Autodesk Fusion 360 part; units mm, degrees
note: some values were not read from the file. Set by a fixed rule: which sketch regions a step uses.
(part 3 of 3)
  line L1632 (31.5149, 83.2092) -> (31.5429, 83.2041)
  line L1633 (34.5916, 83.2488) -> (34.6161, 83.2634)
  line L1634 (34.3999, 83.2001) -> (34.3999, 83.1998)
  line L1635 (34.3999, 83.1998) -> (34.4284, 83.2009)
  line L1636 (34.7988, 83.5713) -> (34.7998, 83.5998)
  line L1637 (34.6396, 83.2796) -> (34.6618, 83.2976)
  line L1638 (31.5429, 83.2041) -> (31.5713, 83.2011)
  line L1639 (31.317, 83.3172) -> (31.3379, 83.2977)
  line L1640 (34.6618, 83.2976) -> (34.6827, 83.317)
  line L1641 (34.7509, 83.4082) -> (34.7637, 83.4337)
  line L1642 (31.5713, 83.2011) -> (31.5999, 83.2001)
  line L1643 (31.4337, 83.2362) -> (31.4601, 83.2253)
  line L1644 (34.4284, 83.2009) -> (34.4568, 83.2039)
  line L1645 (34.7907, 83.5148) -> (34.7958, 83.5429)
  line L1646 (31.4872, 83.2163) -> (31.5149, 83.2092)
  line L1647 (34.7836, 83.4872) -> (34.7907, 83.5148)
  line L1648 (31.2855, 86.2476) -> (31.268, 86.2237)
  line L1649 (34.4568, 83.2039) -> (34.4849, 83.209)
  line L1650 (34.6827, 83.317) -> (34.7022, 83.3379)
  line L1651 (34.5126, 83.2161) -> (34.5397, 83.2251)
  line L1652 (31.4082, 83.249) -> (31.4337, 83.2362)
  line L1653 (31.2488, 83.4083) -> (31.2634, 83.3838)
  line L1654 (31.4601, 83.2253) -> (31.4872, 83.2163)
  line L1655 (34.7201, 83.3601) -> (34.7364, 83.3836)
  line L1656 (34.7746, 83.4601) -> (34.7836, 83.4872)
  line L1657 (34.7022, 83.3379) -> (34.7201, 83.3601)
  line L1658 (31.3836, 83.2635) -> (31.4082, 83.249)
  line L1659 (31.1999, 86.0005) -> (31.1999, 86.0001)
  line L1660 (34.7022, 86.2623) -> (34.6827, 86.2832)
  line L1661 (31.2161, 83.4873) -> (31.2251, 83.4602)
  line L1662 (31.2251, 83.4602) -> (31.236, 83.4339)
  line L1663 (31.4223, 86.3588) -> (31.3962, 86.3446)
  line L1664 (11.2634, 83.3838) -> (11.2797, 83.3603)
  line L1665 (11.2976, 83.3381) -> (11.317, 83.3172)
  line L1666 (11.2161, 83.4873) -> (11.2251, 83.4602)
  line L1667 (14.7022, 86.2623) -> (14.6827, 86.2832)
  line L1668 (14.7958, 86.0573) -> (14.7907, 86.0854)
  line L1669 (11.4771, 86.381) -> (11.4493, 86.3709)
  line L1670 (11.2797, 83.3603) -> (11.2976, 83.3381)
  line L1671 (14.5397, 86.3751) -> (14.5126, 86.3841)
  line L1672 (14.566, 86.3642) -> (14.5397, 86.3751)
  line L1673 (14.7509, 86.192) -> (14.7364, 86.2166)
  line L1674 (14.6396, 86.3206) -> (14.6161, 86.3368)
  line L1675 (14.6161, 86.3368) -> (14.5916, 86.3514)
  line L1676 (14.6618, 86.3026) -> (14.6396, 86.3206)
  line L1677 (11.3254, 86.2913) -> (11.3046, 86.2702)
  line L1678 (11.4223, 86.3588) -> (11.3962, 86.3446)
  line L1679 (14.4568, 86.3963) -> (14.4284, 86.3993)
  line L1680 (14.7988, 86.0289) -> (14.7958, 86.0573)
  line L1681 (14.7836, 86.113) -> (14.7746, 86.1401)
  line L1682 (14.7998, 86.0004) -> (14.7988, 86.0289)
  line L1683 (11.3962, 86.3446) -> (11.3713, 86.3286)
  line L1684 (11.1999, 86.0005) -> (11.1999, 86.0001)
  line L1685 (11.3379, 83.2977) -> (11.3602, 83.2798)
  line L1686 (11.2043, 86.0594) -> (11.201, 86.0299)
  line L1687 (14.7637, 86.1665) -> (14.7509, 86.192)
  line L1688 (11.3713, 86.3286) -> (11.3477, 86.3108)
  line L1689 (14.4284, 86.3993) -> (14.3999, 86.4004)
  line L1690 (14.5126, 86.3841) -> (14.4849, 86.3912)
  line L1691 (14.5916, 86.3514) -> (14.566, 86.3642)
  line L1692 (14.6827, 86.2832) -> (14.6618, 86.3026)
  line L1693 (14.7201, 86.2401) -> (14.7022, 86.2623)
  line L1694 (14.3999, 83.2001) -> (14.3999, 83.1998)
  line L1695 (11.317, 83.3172) -> (11.3379, 83.2977)
  line L1696 (14.5916, 83.2488) -> (14.6161, 83.2634)
  line L1697 (14.7201, 83.3601) -> (14.7364, 83.3836)
  line L1698 (14.7958, 83.5429) -> (14.7988, 83.5713)
  line L1699 (14.6618, 83.2976) -> (14.6827, 83.317)
  line L1700 (11.2009, 83.5715) -> (11.2039, 83.5431)
  line L1701 (14.7998, 83.5998) -> (14.7998, 86.0004)
  line L1702 (14.7988, 83.5713) -> (14.7998, 83.5998)
  line L1703 (11.5713, 83.2011) -> (11.5999, 83.2001)
  line L1704 (11.4082, 83.249) -> (11.4337, 83.2362)
  line L1705 (11.2524, 86.1985) -> (11.2387, 86.1723)
  line L1706 (11.564, 86.3987) -> (11.5346, 86.395)
  line L1707 (11.4337, 83.2362) -> (11.4601, 83.2253)
  line L1708 (14.7509, 83.4082) -> (14.7637, 83.4337)
  line L1709 (11.236, 83.4339) -> (11.2488, 83.4083)
  line L1710 (14.6827, 83.317) -> (14.7022, 83.3379)
  line L1711 (11.3602, 83.2798) -> (11.3836, 83.2635)
  line L1712 (14.3999, 86.4002) -> (11.5999, 86.4002)
  line L1713 (11.5149, 83.2092) -> (11.5429, 83.2041)
  line L1714 (14.5397, 83.2251) -> (14.566, 83.236)
  line L1715 (11.4601, 83.2253) -> (11.4872, 83.2163)
  line L1716 (14.7836, 83.4872) -> (14.7907, 83.5148)
  line L1717 (11.2173, 86.1171) -> (11.2097, 86.0885)
  line L1718 (11.5999, 83.2001) -> (14.3999, 83.2001)
  line L1719 (11.2039, 83.5431) -> (11.209, 83.515)
  line L1720 (14.566, 83.236) -> (14.5916, 83.2488)
  line L1721 (11.1999, 86.0004) -> (11.1999, 86.0005)
  line L1722 (11.2488, 83.4083) -> (11.2634, 83.3838)
  line L1723 (11.2387, 86.1723) -> (11.227, 86.1451)
  line L1724 (14.4284, 83.2009) -> (14.4568, 83.2039)
  line L1725 (11.2251, 83.4602) -> (11.236, 83.4339)
  line L1726 (11.3477, 86.3108) -> (11.3254, 86.2913)
  line L1727 (14.6161, 83.2634) -> (14.6396, 83.2796)
  line L1728 (11.5429, 83.2041) -> (11.5713, 83.2011)
  line L1729 (11.268, 86.2237) -> (11.2524, 86.1985)
  line L1730 (11.1999, 83.6) -> (11.2009, 83.5715)
  line L1731 (11.3836, 83.2635) -> (11.4082, 83.249)
  line L1732 (11.201, 86.0299) -> (11.1999, 86.0004)
  line L1733 (14.7022, 83.3379) -> (14.7201, 83.3601)
  line L1734 (14.3999, 86.4004) -> (14.3999, 86.4002)
  line L1735 (11.5999, 86.4002) -> (11.5935, 86.4003)
  line L1736 (14.4849, 83.209) -> (14.5126, 83.2161)
  line L1737 (14.5126, 83.2161) -> (14.5397, 83.2251)
  line L1738 (11.3046, 86.2702) -> (11.2855, 86.2476)
  line L1739 (14.7907, 83.5148) -> (14.7958, 83.5429)
  line L1740 (14.4568, 83.2039) -> (14.4849, 83.209)
  line L1741 (14.6396, 83.2796) -> (14.6618, 83.2976)
  line L1742 (14.7637, 83.4337) -> (14.7746, 83.4601)
  line L1743 (11.4493, 86.3709) -> (11.4223, 86.3588)
  line L1744 (11.5346, 86.395) -> (11.5056, 86.3891)
  line L1745 (11.5056, 86.3891) -> (11.4771, 86.381)
  line L1746 (11.2097, 86.0885) -> (11.2043, 86.0594)
  line L1747 (11.227, 86.1451) -> (11.2173, 86.1171)
  line L1748 (14.3999, 83.1998) -> (14.4284, 83.2009)
  line L1749 (11.1999, 86.0001) -> (11.1999, 83.6)
  line L1750 (11.4872, 83.2163) -> (11.5149, 83.2092)
  line L1751 (14.7746, 83.4601) -> (14.7836, 83.4872)
  line L1752 (14.7364, 83.3836) -> (14.7509, 83.4082)
  line L1753 (11.2855, 86.2476) -> (11.268, 86.2237)
  line L1754 (11.209, 83.515) -> (11.2161, 83.4873)
  line L1755 (14.7364, 86.2166) -> (14.7201, 86.2401)
  line L1756 (11.5935, 86.4003) -> (11.564, 86.3987)
  line L1757 (14.7746, 86.1401) -> (14.7637, 86.1665)
  line L1758 (14.7907, 86.0854) -> (14.7836, 86.113)
  line L1759 (14.4849, 86.3912) -> (14.4568, 86.3963)
  circle A286 centre (73.2167, 97.5019) radius 0.5715
  circle A287 centre (73.2167, 94.9619) radius 0.5715
  circle A288 centre (70.6767, 94.9619) radius 0.5715
  circle A289 centre (70.6767, 97.5019) radius 0.5715
  circle A290 centre (2.7501, 82.0094) radius 0.1525
  circle A291 centre (4.1397, 72.1394) radius 0.1525
  circle A292 centre (55.3625, 4.8512) radius 0.1525
  circle A293 centre (83.4765, 37.5893) radius 0.1525
  circle A294 centre (84.9014, 37.0879) radius 0.1525
  circle A295 centre (85.5502, 48.3719) radius 0.1525
  circle A296 centre (1.2499, 56.5799) radius 0.1525
  circle A297 centre (1.2629, 36.6652) radius 0.1525
  circle A298 centre (1.2629, 17.0602) radius 0.1525
  circle A299 centre (15.4999, 3.6609) radius 0.1525
  circle A300 centre (82.4298, 9.7066) radius 0.1525
  circle A301 centre (81.87, 25.6347) radius 0.1525
  circle A302 centre (85.5502, 29.0599) radius 0.1525
  circle A303 centre (76.9604, 65.003) radius 0.1525
  circle A304 centre (84.3142, 65.0886) radius 0.1525
  circle A305 centre (55.4999, 94.2799) radius 0.1525
  circle A306 centre (71.8054, 89.6287) radius 0.1525
  circle A307 centre (28.4125, 5.746) radius 0.1525
  circle A308 centre (49.3993, 1.2499) radius 0.1525
  circle A309 centre (17.4168, 5.746) radius 0.1525
  circle A310 centre (1.59, 9.3917) radius 0.1525
  circle A311 centre (6.1252, 12.2731) radius 0.1525
  circle A312 centre (15.459, 4.683) radius 0.1525
  circle A313 centre (36.6005, 2.4468) radius 0.1525
  circle A314 centre (76.6005, 1.2499) radius 0.1525
  circle A315 centre (50.1026, 3.6355) radius 0.1525
  circle A316 centre (86.3874, 68.7488) radius 0.1525
  circle A317 centre (84.05, 69.3995) radius 0.1525
  line L1760 (-10.2, 110.2) -> (97.2, 110.2)
  line L1761 (97.2, 110.2) -> (97.2, -10.2)
  line L1762 (97.2, -10.2) -> (-10.2, -10.2)
  line L1763 (-10.2, -10.2) -> (-10.2, 110.2)
  constraint horizontal L1760
  constraint vertical L1761
  constraint horizontal L1762
  constraint vertical L1763
extrude "Extrude3" add sketch "PCB_hackpad_2026-02-28" 1 faces at (-4.0758, 13, -66.7333) along normal blind 3 separate body contours L0 L1 L2 L3 L200 L201 L202 L204 L205 L206 L207 L212 L213 L214 L215 L216 L217 L218 L220 L221 L222 | L3 L181 L202 L203 L216 L219 L220 L222 | L181 L200 L202 L222 | L181 L202 L203 L222 | L181 L216 L219 L220 | L181 L216 L218 L220 | L181 L200 L201 L222 | L181 L201 L203 L222 | L181 L217 L219 L220 | L181 L217 L218 L220 | L181 L201 L203 L204 L207 L213 L214 L217 L219 L220 L221 L222 | L204 L205 L206 L207 L221 L222 | L204 L207 L221 L222 | L213 L214 L220 L221 | L212 L213 L214 L215 L220 L221 | L36 L37 L38 L39 | L40 L41 L42 L43 | L44 L45 L46 L47 | L48 L49 L50 L51 | L52 L53 L54 L55 | L56 L57 L58 L59 | L60 L61 L62 L63 | L64 L65 L66 L67 | L68 L69 L70 L71 | L72 L73 L74 L75 | L76 L77 L78 L79 | L80 L81 L82 L83 | L84 L85 L86 L87 | L88 L89 L90 L91 | L92 L93 L94 L95 | L96 L97 L98 L99 A87 A169 | L99 A87 A169 A247 | L99 A87 A169 A247 | L99 A247 | L99 A247 | A0 | A1 | A2 | A3 | A4 | A5 | A6 | A7 | A8 | A9 | A10 | A11 | A12 | A13 | A14 | A15 | L101 L102 L103 L104 | L106 L107 L108 L109 | L111 L112 L113 L114 | L116 L117 L118 L119 | L121 L122 L123 L124 | L126 L127 L128 L129 | L131 L132 L133 L134 | L136 L137 L138 L139 | L141 L142 L143 L144 | L146 L147 L148 L149 | L151 L152 L153 L154 | L156 L157 L158 L159 | L161 L162 L163 L164 | L166 L167 L168 L169 | L171 L172 L173 L174 A268 | L173 A268 A304 | L173 A268 A304 | L173 A304 | L173 A304 | L176 L177 L178 L179 | L208 L209 L210 L211 | A16 A94 | A17 A95 | A18 A96 | A19 A97 | A20 A98 | A21 A99 | A22 A100 | A23 A101 | A24 A102 | A25 A103 | A26 A104 | A27 A105 | A28 A106 | A29 A107 | A30 A108 | A31 A109 | A32 A110 | A33 A111 | A34 A112 | A35 A113 | A36 A114 | A37 A115 | A38 A116 | A39 A117 | A40 A118 | A41 A119 | A42 A120 | A43 A121 | A44 A122 | A45 A123 | A46 A124 | A47 A125 | A48 A126 | A49 A127 | A50 A128 | A51 A129 | A52 A130 | A53 A131 | A54 A132 | A55 A133 | A56 A134 | A57 A135 | A58 A136 | A59 A137 | A60 A138 | A61 A139 | A62 A140 | A63 A141 | A64 A142 | A65 A143 | A66 A144 | A67 A145 | A68 A146 | A69 A147 | A70 A148 | A71 A149 | A72 A150 | A73 A151 | A74 A152 | A75 A153 | A76 A154 | A77 A155 | A78 A156 | A79 A157 | A80 A162 | A81 A163 | A82 A164 | A83 A165 | A84 A166 | A85 A167 | A86 A168 | A88 A170 | A89 A171 | A90 A172 | A91 A173 | A92 A174 | A93 A175 | A158 | A159 | A160 | A161 | A176 | A177 | A178 | A179 | A180 | A181 | A182 | A183 | A184 | A185 | A186 | A187 | A188 | A189 | A190 | A191 | A192 | A193 | A194 | A195 | A196 | A197 | A198 | A199 | A200 | A201 | A202 | A203 | A204 | A205 | A206 | A207 | A208 | A209 | A210 | A211 | A212 | A213 | A214 | A215 | A216 | A217 | A218 | A219 | A220 | A221 | A222 | A223 | A224 | A225 | A226 | A227 | A228 | A229 | A230 | A231 | A232 | A233 | A234 | A235 | A236 | A237 | A238 | A239 | A240 | A241 | A242 | A243 | A244 | A245 | A246 | A248 | A249 | A250 | A251 | A252 | A253 | A254 | A255 | A256 | A257 | A258 | A259 | A260 | A261 | A262 | A263 | A264 | A265 | A266 | A267 | A269 | A270 | A271 | A272 | A273 | A274 | A275 | A276 | A277 | A278 | A279 | A280 | A281 | A282 | A283 | A284 | A285 | L224 L225 L226 L227 L228 L229 L230 L231 L232 L233 L234 L236 L237 L238 L239 L240 L241 L242 L243 L244 L245 L246 L247 L248 L249 L250 L251 L252 L253 L254 L255 L256 L257 L258 L259 L260 L262 L263 L265 L266 L268 L269 L270 L271 L272 L273 L274 L275 L276 L277 L278 L279 L280 L281 L282 L283 L284 L285 L286 L287 L288 L289 L290 L291 L292 L293 L294 L295 L296 L297 L298 L299 L300 L301 L302 L303 L304 L305 L306 L307 L308 L309 L310 L311 L312 L313 L314 L315 L316 L317 L318 L319 | L320 L321 L322 L323 L324 L326 L327 L328 L329 L330 L331 L332 L333 L334 L335 L336 L337 L338 L339 L340 L341 L342 L343 L344 L345 L346 L347 L348 L349 L350 L351 L352 L353 L354 L355 L356 L357 L358 L359 L360 L361 L362 L363 L364 L365 L366 L367 L368 L369 L370 L371 L373 L374 L375 L376 L377 L378 L379 L380 L381 L382 L383 L384 L385 L386 L389 L390 L391 L392 L393 L394 L395 L396 L397 L398 L399 L400 L401 L402 L403 L404 L405 L406 L407 L408 L409 L410 L411 L412 L413 L414 L415 | L416 L417 L418 L419 L420 L421 L422 L423 L424 L425 L426 L428 L429 L431 L432 L433 L434 L435 L436 L437 L438 L439 L440 L441 L442 L443 L444 L445 L446 L447 L448 L449 L450 L451 L452 L453 L454 L455 L456 L457 L458 L459 L460 L461 L462 L463 L464 L465 L466 L468 L470 L471 L472 L473 L474 L475 L476 L477 L478 L479 L480 L481 L482 L483 L484 L485 L486 L487 L488 L489 L490 L491 L492 L493 L494 L495 L496 L497 L498 L499 L500 L501 L502 L503 L504 L505 L506 L507 L508 L509 L510 L511 | L512 L513 L514 L515 L516 L517 L518 L519 L520 L521 L522 L523 L524 L525 L526 L527 L528 L529 L530 L531 L532 L533 L534 L535 L536 L537 L538 L539 L540 L542 L543 L544 L545 L546 L547 L548 L549 L550 L551 L552 L553 L554 L555 L556 L557 L558 L559 L560 L561 L562 L563 L564 L565 L566 L567 L568 L569 L571 L572 L573 L574 L575 L576 L577 L578 L579 L580 L581 L582 L583 L584 L585 L586 L587 L589 L590 L591 L592 L593 L594 L595 L596 L598 L599 L600 L601 L602 L603 L604 L605 L606 L607 | L608 L609 L610 L611 L612 L613 L614 L615 L616 L617 L618 L619 L620 L621 L622 L623 L624 L625 L626 L627 L628 L629 L630 L631 L632 L633 L634 L636 L637 L638 L639 L640 L641 L642 L643 L644 L645 L647 L648 L649 L650 L651 L652 L654 L655 L656 L657 L658 L659 L660 L661 L662 L663 L664 L665 L666 L667 L668 L669 L670 L671 L672 L673 L674 L675 L676 L677 L678 L679 L680 L681 L683 L684 L685 L686 L687 L688 L689 L690 L691 L692 L693 L694 L695 L696 L697 L698 L699 L700 L701 L702 L703 | L704 L705 L706 L707 L708 L709 L710 L711 L712 L713 L714 L715 L716 L717 L718 L719 L720 L721 L722 L723 L724 L725 L726 L727 L729 L730 L731 L732 L733 L734 L735 L738 L739 L740 L741 L742 L743 L744 L745 L746 L747 L748 L749 L751 L752 L753 L754 L755 L756 L757 L758 L759 L760 L761 L762 L763 L764 L765 L766 L767 L768 L769 L770 L771 L772 L773 L774 L775 L776 L777 L778 L779 L780 L781 L782 L783 L784 L785 L786 L787 L788 L789 L790 L791 L792 L793 L794 L795 L796 L797 L798 L799 | L800 L801 L802 L803 L804 L805 L806 L807 L808 L809 L811 L812 L813 L814 L815 L816 L817 L818 L819 L820 L821 L822 L823 L824 L825 L826 L827 L828 L829 L830 L831 L832 L833 L834 L835 L836 L837 L838 L839 L840 L841 L842 L843 L844 L845 L846 L847 L848 L849 L850 L851 L852 L853 L854 L855 L856 L857 L858 L859 L860 L861 L862 L863 L865 L866 L867 L868 L869 L870 L871 L872 L873 L874 L875 L876 L877 L878 L879 L880 L881 L883 L884 L885 L886 L887 L888 L889 L890 L891 L892 L894 L895 | L896 L897 L898 L899 L900 L901 L902 L903 L904 L905 L906 L907 L908 L910 L911 L912 L913 L914 L915 L916 L917 L918 L919 L920 L921 L922 L924 L925 L926 L927 L928 L929 L930 L931 L932 L933 L934 L935 L936 L937 L938 L939 L940 L941 L942 L943 L944 L945 L946 L947 L948 L949 L950 L951 L952 L953 L954 L955 L956 L957 L958 L960 L961 L962 L963 L964 L965 L966 L967 L968 L969 L970 L971 L972 L974 L975 L976 L977 L978 L979 L980 L981 L982 L983 L984 L985 L986 L987 L988 L989 L990 L991 | L992 L993 L994 L995 L996 L997 L998 L999 L1000 L1001 L1002 L1003 L1004 L1005 L1006 L1007 L1008 L1009 L1010 L1011 L1012 L1013 L1014 L1015 L1016 L1018 L1019 L1020 L1021 L1022 L1023 L1024 L1026 L1027 L1029 L1030 L1031 L1032 L1033 L1034 L1035 L1036 L1037 L1038 L1039 L1040 L1041 L1042 L1044 L1045 L1046 L1047 L1048 L1049 L1050 L1051 L1052 L1053 L1054 L1055 L1056 L1057 L1058 L1059 L1060 L1061 L1062 L1063 L1064 L1065 L1066 L1067 L1068 L1069 L1070 L1071 L1072 L1073 L1074 L1075 L1076 L1077 L1078 L1079 L1080 L1081 L1082 L1083 L1084 L1085 L1086 L1087 | L1089 L1090 L1091 L1092 L1093 L1094 L1095 L1096 L1097 L1098 L1099 L1100 L1101 L1102 L1103 L1104 L1105 L1106 L1107 L1108 L1110 L1111 L1112 L1113 L1114 L1115 L1116 L1118 L1119 L1120 L1121 L1122 L1123 L1124 L1125 L1126 L1127 L1128 L1129 L1130 L1131 L1132 L1133 L1134 L1135 L1136 L1137 L1138 L1139 L1140 L1141 L1142 L1143 L1144 L1145 L1146 L1147 L1148 L1149 L1150 L1151 L1153 L1154 L1155 L1156 L1157 L1158 L1159 L1160 L1161 L1162 L1163 L1164 L1165 L1166 L1167 L1168 L1169 L1170 L1171 L1172 L1173 L1174 L1175 L1176 L1177 L1178 L1179 L1180 L1181 L1182 L1183 | L1184 L1185 L1186 L1187 L1188 L1189 L1190 L1191 L1192 L1193 L1194 L1195 L1196 L1197 L1198 L1199 L1200 L1201 L1202 L1203 L1204 L1205 L1206 L1207 L1208 L1209 L1210 L1211 L1212 L1213 L1214 L1215 L1216 L1217 L1218 L1219 L1220 L1222 L1223 L1224 L1225 L1226 L1227 L1228 L1229 L1230 L1231 L1232 L1233 L1234 L1235 L1236 L1237 L1238 L1239 L1240 L1241 L1242 L1243 L1244 L1245 L1246 L1247 L1248 L1249 L1250 L1251 L1253 L1254 L1255 L1256 L1257 L1258 L1259 L1260 L1263 L1264 L1265 L1266 L1267 L1268 L1269 L1270 L1271 L1272 L1273 L1274 L1275 L1276 L1277 L1278 L1279 | L1280 L1281 L1282 L1283 L1284 L1285 L1286 L1287 L1288 L1291 L1292 L1293 L1294 L1295 L1296 L1297 L1298 L1299 L1300 L1301 L1302 L1303 L1304 L1305 L1306 L1307 L1308 L1309 L1310 L1311 L1312 L1313 L1314 L1315 L1316 L1317 L1318 L1320 L1321 L1323 L1324 L1325 L1326 L1327 L1328 L1329 L1330 L1331 L1332 L1333 L1334 L1335 L1336 L1337 L1338 L1339 L1340 L1341 L1342 L1343 L1344 L1345 L1346 L1347 L1348 L1349 L1350 L1351 L1352 L1353 L1354 L1355 L1356 L1357 L1358 L1359 L1360 L1361 L1362 L1363 L1364 L1365 L1366 L1367 L1368 L1369 L1370 L1371 L1372 L1373 L1374 L1375 | L1376 L1377 L1378 L1379 L1380 L1381 L1382 L1383 L1384 L1385 L1386 L1387 L1388 L1389 L1390 L1391 L1392 L1393 L1394 L1395 L1397 L1398 L1399 L1400 L1402 L1403 L1404 L1405 L1406 L1407 L1408 L1409 L1410 L1411 L1412 L1413 L1414 L1415 L1416 L1417 L1418 L1419 L1420 L1421 L1422 L1423 L1424 L1425 L1426 L1428 L1430 L1431 L1432 L1433 L1434 L1435 L1436 L1437 L1438 L1439 L1440 L1441 L1442 L1443 L1444 L1445 L1446 L1447 L1448 L1449 L1450 L1451 L1452 L1453 L1454 L1455 L1456 L1457 L1458 L1459 L1460 L1461 L1462 L1463 L1464 L1465 L1466 L1467 L1468 L1469 L1470 L1471 | L1472 L1473 L1474 L1475 L1477 L1478 L1479 L1480 L1481 L1482 L1483 L1484 L1485 L1486 L1487 L1488 L1489 L1490 L1491 L1492 L1493 L1494 L1495 L1496 L1497 L1498 L1499 L1500 L1501 L1502 L1503 L1504 L1505 L1506 L1507 L1508 L1509 L1510 L1511 L1512 L1513 L1514 L1515 L1516 L1517 L1518 L1519 L1520 L1522 L1523 L1524 L1525 L1526 L1527 L1528 L1531 L1532 L1533 L1534 L1535 L1536 L1537 L1538 L1539 L1540 L1541 L1542 L1543 L1544 L1545 L1546 L1547 L1548 L1549 L1550 L1551 L1552 L1553 L1554 L1555 L1556 L1557 L1558 L1559 L1560 L1561 L1562 L1563 L1564 L1565 L1566 L1567 | L1568 L1569 L1570 L1571 L1572 L1573 L1574 L1575 L1576 L1577 L1578 L1579 L1580 L1581 L1582 L1584 L1585 L1586 L1587 L1588 L1589 L1590 L1592 L1593 L1594 L1595 L1596 L1597 L1598 L1599 L1600 L1601 L1602 L1603 L1604 L1605 L1606 L1607 L1608 L1609 L1610 L1611 L1612 L1613 L1614 L1615 L1616 L1617 L1618 L1619 L1620 L1621 L1622 L1623 L1624 L1625 L1626 L1627 L1628 L1629 L1630 L1631 L1632 L1633 L1635 L1636 L1637 L1638 L1639 L1640 L1641 L1642 L1643 L1644 L1645 L1646 L1647 L1648 L1649 L1650 L1651 L1652 L1653 L1654 L1655 L1656 L1657 L1658 L1660 L1661 L1662 L1663 | L1664 L1665 L1666 L1667 L1668 L1669 L1670 L1671 L1672 L1673 L1674 L1675 L1676 L1677 L1678 L1679 L1680 L1681 L1682 L1683 L1685 L1686 L1687 L1688 L1689 L1690 L1691 L1692 L1693 L1695 L1696 L1697 L1698 L1699 L1700 L1701 L1702 L1703 L1704 L1705 L1706 L1707 L1708 L1709 L1710 L1711 L1712 L1713 L1714 L1715 L1716 L1717 L1718 L1719 L1720 L1722 L1723 L1724 L1725 L1726 L1727 L1728 L1729 L1730 L1731 L1732 L1733 L1735 L1736 L1737 L1738 L1739 L1740 L1741 L1742 L1743 L1744 L1745 L1746 L1747 L1748 L1749 L1750 L1751 L1752 L1753 L1754 L1755 L1756 L1757 L1758 L1759 | A286 | A287 | A288 | A289 | A290 | A291 | A292 | A293 | A294 | A295 | A296 | A297 | A298 | A299 | A300 | A301 | A302 | A303 | A305 | A306 | A307 | A308 | A309 | A310 | A311 | A312 | A313 | A314 | A315 | A316 | A317 | L1760 L1761 L1762 L1763 on bodies 1 makes body 2
extrude "Extrude4" cut sketch "PCB_hackpad_2026-02-28" along normal blind 20 contours L36 L37 L38 L39 | L40 L41 L42 L43 | L44 L45 L46 L47 | L48 L49 L50 L51 | L52 L53 L54 L55 | L56 L57 L58 L59 | L60 L61 L62 L63 | L64 L65 L66 L67 | L68 L69 L70 L71 | L72 L73 L74 L75 | L76 L77 L78 L79 | L80 L81 L82 L83 | L84 L85 L86 L87 | L88 L89 L90 L91 | L92 L93 L94 L95 | L96 L97 L98 L99 A87 A169 | L99 A87 A169 A247 | L99 A247 | A271 | A273 | A275 | A307 | A309 | A311 picked at (79.5349, 80.9791) picked at (79.5462, 80.9875) bodies 2
extrude "Extrude5" cut sketch "Sketch1" along normal blind 100 contours A0 | A1 | A2 | A3 bodies 2
sketch "Sketch3" plane through (0, 0, -110.2) normal (0, 0, -1) x (-1, 0, 0)
  line L0 (-97.2, 0) -> (10.2, 0)
  line L1 (10.2, 0) -> (10.2, 13)
  line L2 (10.2, 13) -> (-97.2, 13)
  line L3 (-97.2, 13) -> (-97.2, 0)
  line L4 (-79.1024, 3) -> (-64.1024, 3)
  line L5 (-64.1024, 3) -> (-64.1024, 9)
  line L6 (-64.1024, 9) -> (-79.1024, 9)
  line L7 (-79.1024, 9) -> (-79.1024, 3)
  line L8 (-97.2, 0) -> (10.2, 0)
  dimension "d27" = 3
  dimension "d28" = 15
  dimension "d29" = 6
  constraint horizontal L4
  constraint vertical L5
  constraint horizontal L6
  constraint vertical L7
  measures "d27" distance of L4 L8
  measures "d28" distance of L5.end L6.end
  measures "d29" distance of L4.end L5.end
extrude "Extrude6" cut sketch "Sketch3" against normal blind 12 contours L4 L5 L6 L7 bodies 1
fillet "Fillet1" radius 4.5 8 edges at (-10.2, 6.5, 10.2) (97.2, 6.5, 10.2) (97.2, 6.5, -110.2) (-10.2, 6.5, -110.2) (-10.2, 14.5, 10.2) (97.2, 14.5, 10.2) (97.2, 14.5, -110.2) (-10.2, 14.5, -110.2) on bodies 1 2
fillet "Fillet2" radius 1.5 16 edges at (43.5, 0, 10.2) (95.882, 0, 8.882) (97.2, 0, -50) (95.882, 0, -108.882) (43.5, 0, -110.2) (-8.882, 0, -108.882) (-10.2, 0, -50) (-8.882, 0, 8.882) (-8.882, 16, 8.882) (43.5, 16, 10.2) (95.882, 16, 8.882) (97.2, 16, -50) (95.882, 16, -108.882) (43.5, 16, -110.2) (-8.882, 16, -108.882) (-10.2, 16, -50) on bodies 1 2
fillet "Fillet3" radius 0.5 128 edges at (5.3349, 14.5, -80.9901) (13.1349, 16, -80.9901) (5.3349, 16, -73.1901) (13.1349, 16, -65.3901) (5.3349, 14.5, -65.3901) (20.9348, 14.5, -80.9901) (20.9348, 16, -73.1901) (20.9348, 14.5, -65.3901) (25.3349, 14.5, -80.9901) (25.3349, 16, -73.1901) (33.1349, 16, -80.9901) (25.3349, 14.5, -65.3901) (33.1349, 16, -65.3901) (40.9348, 14.5, -65.3901) (40.9348, 16, -73.1901) (40.9348, 14.5, -80.9901) (45.3349, 14.5, -65.3901) (45.3349, 16, -73.1901) (53.1349, 16, -65.3901) (53.1349, 16, -80.9901) (45.3349, 14.5, -80.9901) (60.9348, 14.5, -65.3901) (60.9348, 16, -73.1901) (60.9348, 14.5, -80.9901) (73.1349, 16, -80.9901) (65.3349, 16, -73.1901) (65.3349, 14.5, -80.9901) (65.3349, 14.5, -65.3901) (73.1349, 16, -65.3901) (80.9348, 14.5, -65.3901) (80.9348, 16, -73.1901) (80.9348, 14.5, -80.9901) (5.3349, 14.5, -60.9901) (13.1349, 16, -60.9901) (5.3349, 16, -53.1901) (5.3349, 14.5, -45.3901) (13.1349, 16, -45.3901) (20.9348, 16, -53.1901) (20.9348, 14.5, -45.3901) (20.9348, 14.5, -60.9901) (25.3349, 14.5, -60.9901) (25.3349, 16, -53.1901) (33.1349, 16, -60.9901) (40.9348, 14.5, -60.9901) (40.9348, 16, -53.1901) (33.1349, 16, -45.3901) (25.3349, 14.5, -45.3901) (40.9348, 14.5, -45.3901) (45.3349, 16, -53.1901) (53.1349, 16, -60.9901) (45.3349, 14.5, -60.9901) (45.3349, 14.5, -45.3901) (53.1349, 16, -45.3901) (60.9348, 16, -53.1901) (60.9348, 14.5, -60.9901) (60.9348, 14.5, -45.3901) (65.3349, 14.5, -60.9901) (73.1349, 16, -60.9901) (65.3349, 16, -53.1901) (65.3349, 14.5, -45.3901) (73.1349, 16, -45.3901) (80.9348, 14.5, -45.3901) (80.9348, 16, -53.1901) (80.9348, 14.5, -60.9901) (5.3349, 14.5, -40.9901) (13.1349, 16, -40.9901) (5.3349, 16, -33.1901) (5.3349, 14.5, -25.3901) (13.1349, 16, -25.3901) (20.9348, 16, -33.1901) (20.9348, 14.5, -40.9901) (20.9348, 14.5, -25.3901) (33.1349, 16, -25.3901) (25.3349, 16, -33.1901) (25.3349, 14.5, -40.9901) (33.1349, 16, -40.9901) (25.3349, 14.5, -25.3901) (40.9348, 14.5, -40.9901) (40.9348, 16, -33.1901) (40.9348, 14.5, -25.3901) (45.3349, 14.5, -25.3901) (45.3349, 14.5, -40.9901) (45.3349, 16, -33.1901) (53.1349, 16, -40.9901) (53.1349, 16, -25.3901) (60.9348, 14.5, -25.3901) (60.9348, 14.5, -40.9901) (60.9348, 16, -33.1901) (65.3349, 16, -33.1901) (65.3349, 14.5, -40.9901) (73.1349, 16, -40.9901) (65.3349, 14.5, -25.3901) (73.1349, 16, -25.3901) (80.9348, 16, -33.1901) (80.9348, 14.5, -40.9901) (80.9348, 14.5, -25.3901) (5.3349, 14.5, -20.9901) (5.3349, 16, -13.1901) (13.1349, 16, -20.9901) (13.1349, 16, -5.3901) (20.9348, 16, -13.1901) (20.9348, 14.5, -20.9901) (5.3349, 14.5, -5.3901) (20.9348, 14.5, -5.3901) (25.3349, 14.5, -5.3901) (25.3349, 16, -13.1901) (25.3349, 14.5, -20.9901) (33.1349, 16, -20.9901) (33.1349, 16, -5.3901) (40.9348, 14.5, -5.3901) (40.9348, 16, -13.1901) (40.9348, 14.5, -20.9901) (45.3349, 16, -13.1901) (45.3349, 14.5, -20.9901) (53.1349, 16, -20.9901) (60.9348, 14.5, -5.3901) (53.1349, 16, -5.3901) (45.3349, 14.5, -5.3901) (60.9348, 14.5, -20.9901) (60.9348, 16, -13.1901) (65.3349, 16, -13.1901) (73.1349, 16, -5.3901) (65.3349, 14.5, -5.3901) (65.3349, 14.5, -20.9901) (73.1349, 16, -20.9901) (80.9348, 14.5, -5.3901) (80.9348, 16, -13.1901) (80.9348, 14.5, -20.9901) on bodies 2
extrude "Extrude8" add sketch "Sketch1" along normal blind 1.6 from surface at 4 separate body contours L0 L1 L2 L3 makes body 3
fillet "Fillet4" radius 0.25 8 edges at (64.1024, 3, -105.2) (71.6024, 3, -110.2) (64.1024, 6, -110.2) (64.1024, 9, -105.2) (71.6024, 9, -110.2) (79.1024, 9, -105.2) (79.1024, 6, -110.2) (79.1024, 3, -105.2) on bodies 1
equation "d8 = d5"
equation "d9 = d7"
equation "d10 = d6"
equation "d11 = d5"
equation "d12 = d6"
equation "d13 = d7"
equation "d14 = d5"
equation "d15 = d6"
equation "d16 = d7"
named bodies: "Bottom", "Top", "PCB"
